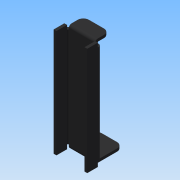
# Autodesk Inventor part: крепление бабины
Saved by Autodesk Inventor 2017 (Build 210142000, 142)
## iProperties
Part Number: крепление бабины
Material: Типовые
Document SubType Name: Modeling
Designer: Max
Mass: 7.11938 g
Surface Area: 77.0009 cm^2
Volume: 7.11938 cm^3
Density: 1 g/cm^3
Appearance: Резина — черная
Author: Max
Autodesk Inventor part; units mm, degrees
ref_plane "YZ Plane" through (0, 0, 0) normal (1, 0, 0) x (0, 1, 0)
ref_plane "XZ Plane" through (0, 0, 0) normal (0, 1, 0) x (-1, 0, 0)
ref_plane "XY Plane" through (0, 0, 0) normal (0, 0, 1) x (1, 0, 0)
sketch "Эскиз1" plane through (0, 0, 0) normal (0, 0, 1) x (1, 0, 0)
  line L0 (0, 0) -> (0, 11.2754) construction
  line L1 (0, 0) -> (-17.0842, 0) construction
  line L2 (-12.15, 0) -> (12.15, 0)
  line L3 (12.15, 0) -> (12.15, 10.3)
  line L4 (12.15, 10.3) -> (-12.15, 10.3)
  line L5 (-12.15, 10.3) -> (-12.15, 0)
  line L6 (-10.15, 0) -> (10.15, 0)
  line L7 (10.15, 0) -> (10.15, 8.3)
  line L8 (10.15, 8.3) -> (-10.15, 8.3)
  line L9 (-10.15, 8.3) -> (-10.15, 0)
  dimension "d0" = 2
  dimension "d1" = 2
  dimension "d2" = 2
  dimension "d3" = 24.3
  dimension "d4" = 10.3
  constraints: 20 end point, 4 parallel, 3 horizontal, 2 perpendicular, 2 point on line, 1 vertical, 1 other
  measures "d0" distance between parallel lines of L8 L4
  measures "d1" distance between parallel lines of L5 L9
  measures "d2" distance between parallel lines of L3 L7
  measures "d3" distance between parallel lines of L3 L5
  measures "d4" distance between parallel lines of L2 L4
extrude "Выдавливание1" add sketch "Эскиз1" along normal mid plane 78 contours L5 L4 L3 L2 L7 L8 L9
sketch "Эскиз2" plane through (-12.15, 10.3, -39) normal (0, 1, 0) x (1, 0, 0)
  line L0 (0, 0) -> (24.3, 0) projected
  line L1 (2.65, 0) -> (21.65, 0)
  line L2 (21.65, 0) -> (21.65, -2)
  line L3 (21.65, -2) -> (2.65, -2)
  line L4 (2.65, -2) -> (2.65, 0)
  line L5 (24.3, -78) -> (0, -78) projected
  line L6 (2.65, -78) -> (21.65, -78)
  line L7 (21.65, -78) -> (21.65, -76)
  line L8 (21.65, -76) -> (2.65, -76)
  line L9 (2.65, -76) -> (2.65, -78)
  line L10 (12.15, -39) -> (12.15, -67.9082) construction
  dimension "d7" = 2
  dimension "d8" = 2
  dimension "d9" = 19
  dimension "d10" = 19
  constraints: 18 end point, 4 parallel, 3 point on line, 2 horizontal, 2 perpendicular, 1 vertical, 3 other
  measures "d7" distance of the line from the sketch origin of L3
  measures "d8" distance between parallel lines of L5 L8
  measures "d9" distance between parallel lines of L2 L4
  measures "d10" distance between parallel lines of L7 L9
extrude "Выдавливание2" add sketch "Эскиз2" along normal blind 8.5 contours L5 L9 L8 L7
extrude "Выдавливание3" add sketch "Эскиз2" along normal blind 18 contours L0 L2 L3 L4
fillet "Сопряжение1" radius 4 4 edges at (9.5, 28.3, -38) (-9.5, 28.3, -38) (-9.5, 18.8, 38) (9.5, 18.8, 38)
sketch "Эскиз3" plane through (-9.5, 10.3, -37) normal (0, 0, 1) x (1, 0, 0)
  line L0 (9.5, -10.3) -> (9.5, 21.9843) construction
  circle A0 centre (9.5, 8) radius 1.6
  line L1 (15, 18) -> (4, 18) projected
  dimension "d16" = 3.2
  dimension "d17" = 10
  constraints: 2 end point, 1 centre point, 1 point on line, 1 vertical
  measures "d16" diameter of A0
  measures "d17" distance from line of L1 A0.centre
extrude "Выдавливание4" cut sketch "Эскиз3" against normal blind 18
sketch "Эскиз4" plane through (0, 0, 39) normal (0, 0, 1) x (1, 0, 0)
  line L0 (12.15, 0) -> (12.15, 10.3) projected
  line L1 (9.5, 10.3) -> (12.15, 10.3)
  line L2 (12.15, 10.3) -> (12.15, 7.7)
  line L3 (12.15, 7.7) -> (9.5, 7.7)
  line L4 (9.5, 7.7) -> (9.5, 10.3)
  line L5 (10.15, 0) -> (12.15, 0) projected
  line L6 (-12.15, 10.3) -> (-9.5, 10.3) projected
  line L7 (-9.5, 10.3) -> (-15.4416, 10.3)
  line L8 (-15.4416, 10.3) -> (-15.4416, 7.7)
  line L9 (-15.4416, 7.7) -> (-9.5, 7.7)
  line L10 (-9.5, 7.7) -> (-9.5, 10.3)
  line L11 (-12.15, 0) -> (-10.15, 0) projected
  point P0 (0, 0)
  dimension "d20" = 7.7
  dimension "d21" = 7.7
  constraints: 16 end point, 4 parallel, 2 horizontal, 2 perpendicular, 1 point on line
  measures "d20" distance between parallel lines of L5 L3
  measures "d21" distance between parallel lines of L11 L9
extrude "Выдавливание5" cut sketch "Эскиз4" against normal blind 3
mirror "Зеркальное отражение1" about plane through (0, 0, 0) normal (0, 0, 1) of "Выдавливание5"
fillet "Сопряжение2" radius 2 4 edges at (0, 8.3, 39) (12.15, 10.3, 0) (-12.15, 10.3, 0) (0, 8.3, -39)
fillet "Сопряжение3" radius 0.5 4 edges at (0, 10.3, -37) (0, 10.3, 37) (10.15, 8.3, 0) (-10.15, 8.3, 0)
